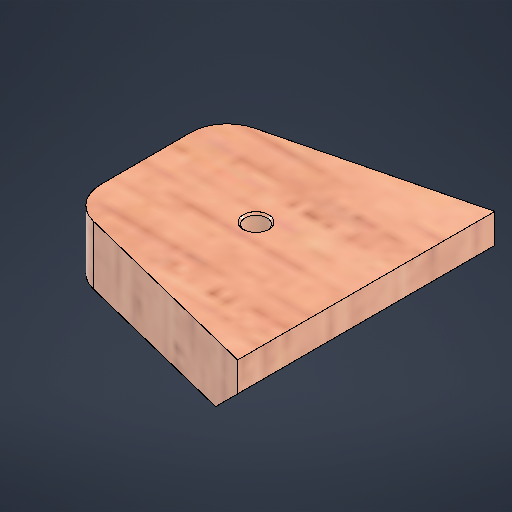
# Autodesk Inventor part: TCSM1-002A
Saved by Autodesk Inventor 2025.3 (Build 293356000, 356)
## iProperties
Created: 2025-08-24
Part Number: TCSM1-002A
Material: Wood (Oak)
Document SubType Name: Modeling
Designer: fablabadmin
Density: 0.76 g/cm^3
Appearance: White Oak - Natural Medium Gloss
Author: fablabadmin
Autodesk Inventor part; units mm, degrees
ref_plane "YZ Plane" through (0, 0, 0) normal (1, 0, 0) x (0, 1, 0)
ref_plane "XZ Plane" through (0, 0, 0) normal (0, 1, 0) x (-1, 0, 0)
ref_plane "XY Plane" through (0, 0, 0) normal (0, 0, 1) x (1, 0, 0)
sketch "Sketch1" plane through (0, 0, 0) normal (0, 1, 0) x (-1, 0, 0)
  line L0 (-15, 17.5) -> (15, 17.5)
  line L1 (15, 17.5) -> (15, -17.5)
  line L2 (15, -17.5) -> (-15, -17.5)
  line L3 (-15, -17.5) -> (-15, 17.5)
  line L4 (-15, 17.5) -> (15, -17.5) construction
  line L5 (15, 17.5) -> (-15, -17.5) construction
  line L6 (15, -10) -> (-15, -17.5)
  line L7 (21, 0) -> (-21, 0) construction
  line L8 (15, 10) -> (-15, 17.5)
  point P0 (0, 0)
  point P1 (0, 0)
  point P2 (15, 10)
  dimension "d1" = 30
  dimension "d2" = 35
  dimension "d19" = 20
  dimension "d20" = 30
  constraints: 16 end point, 2 midpoint, 2 parallel, 2 point on line, 2 symmetric about line, 1 coincident, 1 horizontal, 1 perpendicular
  measures "d1" distance of L1.end L2.end
  measures "d2" distance of L0.end L1.end
  measures "d19" distance of L8.start L6.start
  measures "d20" horizontal distance of L6.end L6.start
extrude "Extrusion1" add sketch "Sketch1" against normal blind 8 contours L8 L1 L6 L3
hole "Hole1" at (0, 0, 0) direction (0, -1, 0) diameter 3 end through all countersink diameter 3.5 countersink angle 90
chamfer "Chamfer1" distance 0.25 angle 45 1 edges at (0, -8, -1.5)
fillet "Fillet1" radius 5 2 edges at (-15, -4, 10) (-15, -4, -10)
chamfer "Chamfer3" distance 4 angle 45 1 edges at (15, -8, 0)
body "Solid1"
